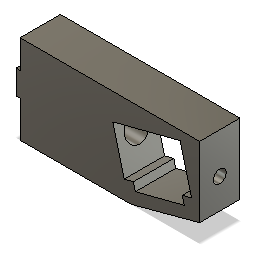
LED-Mount (Autodesk Fusion 360 design; units mm, degrees)
Autodesk Fusion 360 part; units mm, degrees
note: some values were not read from the file. Set by a fixed rule: which sketch regions a step uses.
sketch "Sketch1" plane through (0, 0, 0) normal (0, 0, 1) x (1, 0, 0)
  line L0 (0, 13) -> (44.5, 13)
  line L1 (0, 0) -> (-1, 0)
  line L2 (-1, 0) -> (-1, 6)
  line L3 (-1, 6) -> (0, 6)
  line L4 (0, -9) -> (27.5027, -9)
  line L5 (44.5, 13) -> (44.5, -4.4456)
  line L6 (9.2672, -6.9165) -> (19.8794, -6.9165) construction
  line L7 (25.7993, -4.4556) -> (22.983, 6.4362)
  line L8 (22.983, 6.4362) -> (39.6837, 10.7545)
  line L9 (39.6837, 10.7545) -> (42.5, -0.1373)
  line L10 (0, 13) -> (0, 6)
  line L11 (0, 0) -> (0, -9)
  line L12 (27.5027, -9) -> (28.2069, -8.8113)
  line L13 (27.5027, -9) -> (27.6263, -9) construction
  line L14 (28.5868, -5.749) -> (28.0986, -3.8611)
  line L15 (40.6888, -2.6198) -> (40.2006, -0.7319)
  line L16 (28.0986, -3.8611) -> (25.7993, -4.4556)
  line L17 (40.2006, -0.7319) -> (42.5, -0.1373)
  line L18 (28.5868, -5.749) -> (40.6888, -2.6198)
  line L19 (28.2069, -8.8113) -> (44.5, -4.4456)
  point P0 (28.5868, -5.749)
  dimension "d1" = 44.5
  dimension "d3" = 1
  dimension "d4" = 6
  dimension "d6" = 9
  dimension "d7" = 7
  dimension "d15" = 17.25
  dimension "d25" = 15
  dimension "d26" = 12.5
  dimension "d30" = 2
  dimension "d31" = 105
  dimension "d33" = 2.75
  dimension "d34" = 13.2
  dimension "d35" = 16.9973
  dimension "d38" = 11.25
  measures "d1" distance of L0.start L0.end
  measures "d3" distance of L1.start L1.end
  measures "d4" distance of L1.end L2.end
  measures "d6" distance of L1 L4
  measures "d7" distance of L0 L3
  measures "d15" distance of L7.end L8.end
  measures "d25" angle of L12 L13
  measures "d26" distance of L14 L15
  measures "d30" distance of L5 L9.end
  measures "d31" angle of L5 L12
  measures "d33" distance of L12 L15.start
  measures "d34" distance of L8 L18
  measures "d35" distance of L5 L4.end
  measures "d38" distance of L8 L16
extrude "Extrude1" add sketch "Sketch1" along normal blind 10
sketch "Sketch2" plane through (-1, 0, 0) normal (-1, 0, 0) x (0, 0, 1)
  line L0 (0, 6) -> (0, 0)
  line L1 (0, 0) -> (10, 0)
  line L2 (10, 0) -> (10, 6)
  line L3 (10, 6) -> (0, 6)
  circle A0 centre (5, 3) radius 1.6
  circle A1 centre (5, 3) radius 3
  dimension "d18" = 3.2
  dimension "d19" = 6
  measures "d18" diameter of A0
  measures "d19" diameter of A1
extrude "Extrude2" cut sketch "Sketch2" against normal up to surface (45.5 mm away) contours A0
ref_plane "WorkPlane1" through (26, 3, 5) normal (-1, 0, 0) x (0, 0, 1)
sketch "Sketch3" plane through (26, 3, 2.5) normal (-1, 0, 0) x (0, 0, -1)
  circle A0 centre (-2.5, 0) radius 3
  point P0 (-2.5, 0)
extrude "Extrude3" cut sketch "Sketch3" along normal blind 23
equation "d1 = 27.5 mm + 17 mm"
equation "d23 = 27 mm - 4 mm"
